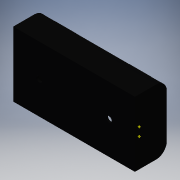
# Autodesk Inventor part: AAHolder
Saved by Autodesk Inventor 2016 (Build 200138000, 138)
## iProperties
Created: 2016-06-11
Part Number: AAHolder
Material: ABS Plastic
Document SubType Name: Modeling
Designer: Tyler
Density: 1.06 g/cm^3
Appearance: Smooth - Black
Author: Tyler
Autodesk Inventor part; units mm, degrees
ref_plane "YZ Plane" through (0, 0, 0) normal (1, 0, 0) x (0, 1, 0)
ref_plane "XZ Plane" through (0, 0, 0) normal (0, 1, 0) x (-1, 0, 0)
ref_plane "XY Plane" through (0, 0, 0) normal (0, 0, 1) x (1, 0, 0)
sketch "Sketch1" plane through (0, 0, 0) normal (1, 0, 0) x (0, 1, 0)
  line L0 (15, 15.25) -> (0, 15.25)
  line L1 (0, 15.25) -> (0, -15.25)
  line L2 (0, -15.25) -> (15, -15.25)
  line L3 (15, -15.25) -> (15, 15.25)
  line L4 (15, 15.25) -> (0, -15.25) construction
  line L5 (0, 15.25) -> (15, -15.25) construction
  point P0 (0, 0)
  point P1 (7.5, 0)
  dimension "d0" = 15
  dimension "d1" = 30.5
  dimension "d2" = 0
  dimension "d3" = 0
  constraints: 12 end point, 2 midpoint, 2 parallel, 1 horizontal, 1 perpendicular
  measures "d0" distance of L1.end L2.end
  measures "d1" distance of L0.end L1.end
  measures "d2" distance from line of point (0, 0) L1
  measures "d3" vertical distance of point (0, 0) point (7.5, 0)
extrude "Extrusion1" add sketch "Sketch1" along normal mid plane 57.2
fillet "Fillet1" radius 5 2 edges at (0, 15, 15.25) (0, 15, -15.25)
sketch "Sketch2" plane through (0, 0, 0) normal (1, 0, 0) x (0, 1, 0)
  arc A0 (10, -15.25) -> (15, -10.25) centre (10, -10.25) ccw projected
  line L0 (15, -10.25) -> (15, 10.25) projected
  arc A1 (15, 10.25) -> (10, 15.25) centre (10, 10.25) ccw projected
  line L1 (10, 15.25) -> (0, 15.25) projected
  line L2 (0, 15.25) -> (0, -15.25) projected
  line L3 (0, -15.25) -> (10, -15.25) projected
  line L4 (1, 14.25) -> (10, 14.25)
  arc A2 (14, 10.25) -> (10, 14.25) centre (10, 10.25) ccw
  line L5 (14, 10.25) -> (14, -10.25)
  arc A3 (10, -14.25) -> (14, -10.25) centre (10, -10.25) ccw
  line L6 (10, -14.25) -> (1, -14.25)
  line L7 (1, -14.25) -> (1, 14.25)
  point P0 (0, 0)
  dimension "d7" = 1
  constraints: 8 end point, 4 point on circle, 2 centre point, 5 other
  measures "d7" distance between parallel lines of L0 L5
extrude "Extrusion2" cut sketch "Sketch2" along normal mid plane 55.2 contours L4 A2 L5 A3 L6 L7
sketch "Sketch3" plane through (-28.6, 15, -10.25) normal (0, 1, 0) x (1, 0, 0)
  line L0 (0, -20.5) -> (0, 0) construction
  line L1 (57.2, -20.5) -> (0, -20.5) construction
  line L2 (57.2, 0) -> (57.2, -20.5) construction
  line L3 (1, 4) -> (1, -24.5)
  line L4 (1, -24.5) -> (6, -24.5)
  line L5 (6, -24.5) -> (6, -21.5)
  line L6 (6, -21.5) -> (16, -21.5)
  line L7 (16, -21.5) -> (16, -24.5)
  line L8 (16, -24.5) -> (41.2, -24.5)
  line L9 (41.2, -24.5) -> (41.2, -21.5)
  line L10 (41.2, -21.5) -> (51.2, -21.5)
  line L11 (51.2, -21.5) -> (51.2, -24.5)
  line L12 (51.2, -24.5) -> (56.2, -24.5)
  line L13 (56.2, -24.5) -> (56.2, 4)
  line L14 (56.2, 4) -> (51.2, 4)
  line L15 (51.2, 4) -> (51.2, 1)
  line L16 (51.2, 1) -> (41.2, 1)
  line L17 (41.2, 1) -> (41.2, 4)
  line L18 (41.2, 4) -> (16, 4)
  line L19 (16, 4) -> (16, 1)
  line L20 (16, 1) -> (6, 1)
  line L21 (6, 1) -> (6, 4)
  line L22 (6, 4) -> (1, 4)
  line L23 (57.2, 5) -> (0, 5) projected
  line L24 (0, -25.5) -> (57.2, -25.5) projected
  point P0 (28.6, -10.25)
  dimension "d10" = 1
  dimension "d11" = 1
  dimension "d12" = 1
  dimension "d13" = 1
  dimension "d14" = 10
  dimension "d15" = 5
  dimension "d16" = 3
  constraints: 40 end point, 14 collinear, 11 parallel, 8 perpendicular
  measures "d10" distance between parallel lines of L0 L3
  measures "d11" distance between parallel lines of L2 L13
  measures "d12" distance between parallel lines of L23 L18
  measures "d13" distance between parallel lines of L24 L8
  measures "d14" distance of L19.end L20.end
  measures "d15" distance of L21.end L3.start
  measures "d16" distance between parallel lines of L18 L20
extrude "Extrusion3" cut sketch "Sketch3" against normal up to next
sketch "Sketch4" plane through (-27.6, 1, 14.25) normal (0, 1, 0) x (1, 0, 0)
  line L0 (0, 0) -> (55.2, 0) projected
  line L1 (55.2, 28.5) -> (0, 28.5) projected
  point P0 (27.6, 14.25)
  point P1 (11.25, 14.25)
  point P2 (43.95, 14.25)
  dimension "d19" = 32.7
  dimension "d20" = 16.35
  dimension "d21" = 14.25
  dimension "d22" = 14.25
  dimension "d23" = 14.25
  measures "d19" distance of point (43.95, 14.25) point (11.25, 14.25)
  measures "d20" distance of point (27.6, 14.25) point (11.25, 14.25)
  measures "d21" distance from line of L1 point (11.25, 14.25)
  measures "d22" distance from line of L0 point (11.25, 14.25)
  measures "d23" distance from line of L1 point (43.95, 14.25)
hole "Hole1" at (-16.35, 1, 0) at (16.35, 1, 0) direction (0, -1, 0) diameter 2.7 end through all
sketch "Sketch5" plane through (-27.6, 0, 0) normal (1, 0, 0) x (0, 0, -1)
  line L0 (14.25, 1) -> (-14.25, 1) projected
  line L1 (-10.25, 15) -> (10.25, 15) projected
  circle A0 centre (7.2, 8.2) radius 1.2755
  line L2 (0, 0) -> (0, 12.8621) construction
  dimension "d31" = 7.2
  dimension "d32" = 7.2
  constraints: 2 end point, 1 centre point, 1 perpendicular
  measures "d31" distance from line of L2 A0.centre
  measures "d32" distance from line of L0 A0.centre
extrude "Extrusion4" add sketch "Sketch5" along normal blind 1
pattern_circular "Circular Pattern1" count 2 over 360 about axis through (0, -10, 0) along (0, 1, 0) of "Extrusion4"
sketch "Sketch6" plane through (28.6, 0, 0) normal (1, 0, 0) x (0, 0, -1)
  circle A0 centre (-2, 2) radius 1
  circle A1 centre (2, 2) radius 1
  line L0 (-14.25, 1) -> (14.25, 1) projected
  point P0 (0, 0)
  dimension "d38" = 2
  dimension "d39" = 2
  dimension "d40" = 2
  dimension "d41" = 2
  constraints: 2 centre point, 2 tangent
  measures "d38" diameter of A0
  measures "d39" diameter of A1
  measures "d40" horizontal distance of A0.centre point (0, 0)
  measures "d41" horizontal distance of point (0, 0) A1.centre
extrude "Extrusion5" cut sketch "Sketch6" against normal blind 0.5
sketch "Sketch7" plane through (28.6, 0, 0) normal (1, 0, 0) x (0, 0, -1)
  circle A0 centre (2, 2) radius 1 projected
sketch "Sketch8" plane through (28.6, 0, 0) normal (1, 0, 0) x (0, 0, -1)
  circle A0 centre (-2, 2) radius 1 projected
equation "\"d13\" = d12"
equation "\"d20\" = 0.5 * d19"
equation "\"d21\" = d22"
equation "\"d23\" = d21"
equation "\"d32\" = d31"
body "Solid1"
